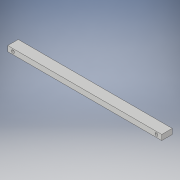
# Autodesk Inventor part: GlyphPlateBackSide
Saved by Autodesk Inventor 2017 (Build 210142000, 142)
## iProperties
Created: 2018-01-27
Part Number: GlyphPlateBackSide
Material: Generic
Document SubType Name: Modeling
Designer: User
Density: 1 g/cm^3
Appearance: Default
Author: User
Autodesk Inventor part; units mm, degrees
ref_plane "YZ Plane" through (0, 0, 0) normal (1, 0, 0) x (0, 1, 0)
ref_plane "XZ Plane" through (0, 0, 0) normal (0, 1, 0) x (-1, 0, 0)
ref_plane "XY Plane" through (0, 0, 0) normal (0, 0, 1) x (1, 0, 0)
sketch "Sketch1" plane through (0, 0, 0) normal (0, 0, 1) x (1, 0, 0)
  line L0 (0, 0) -> (185.8518, 0)
  line L1 (185.8518, 0) -> (185.8518, 6.35)
  line L2 (185.8518, 6.35) -> (0, 6.35)
  line L3 (0, 6.35) -> (0, 0)
  dimension "d0" = 185.8518
  dimension "d1" = 6.35
  constraints: 8 end point, 2 parallel, 1 horizontal, 1 perpendicular
  measures "d0" distance of L2.end L1.end
  measures "d1" distance of L1.end L0.end
extrude "Extrusion1" add sketch "Sketch1" along normal blind 12.7
sketch "Sketch2" plane through (0, 0, 12.7) normal (0, 0, 1) x (1, 0, 0)
  line L0 (0, 6.35) -> (0, 0) projected
  line L1 (0, 3.175) -> (6.35, 3.175)
  line L2 (185.8518, 0) -> (185.8518, 6.35) projected
  line L3 (185.8518, 3.175) -> (179.5018, 3.175)
  circle A0 centre (179.5018, 3.175) radius 1.778
  circle A1 centre (6.35, 3.175) radius 1.778
  dimension "d4" = 6.35
  dimension "d5" = 6.35
  dimension "d6" = 3.556
  dimension "d7" = 3.556
  constraints: 4 end point, 2 centre point, 2 coincident, 2 horizontal, 2 midpoint
  measures "d4" distance of L1.start L1.end
  measures "d5" distance of L3.start L3.end
  measures "d6" diameter of A0
  measures "d7" diameter of A1
extrude "Extrusion2" cut sketch "Sketch2" against normal blind 12.7
body "Solid1"
